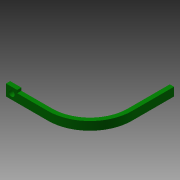
# Autodesk Inventor part: BackNetHookLeft
Saved by Autodesk Inventor 2014 SP1 (Build 180222100, 222)
## iProperties
Created: 2017-01-20
Part Number: BackNetHookLeft
Material: Generic
Document SubType Name: Modeling
Designer: danielsikar
Density: 1 g/cm^3
Appearance: Dark Green
Author: danielsikar
Autodesk Inventor part; units mm, degrees
ref_plane "YZ Plane" through (0, 0, 0) normal (1, 0, 0) x (0, 1, 0)
ref_plane "XZ Plane" through (0, 0, 0) normal (0, 1, 0) x (-1, 0, 0)
ref_plane "XY Plane" through (0, 0, 0) normal (0, 0, 1) x (1, 0, 0)
sketch "Sketch1" plane through (0, 0, 0) normal (0, 0, 1) x (1, 0, 0)
  line L0 (0, 0) -> (60, 0) construction
  line L1 (60, 0) -> (60, 60) construction
  line L2 (60, 60) -> (0, 60) construction
  line L3 (0, 3) -> (0, 0)
  line L4 (57, 60) -> (60, 60)
  line L5 (60, 60) -> (60, 30)
  line L6 (60, 0) -> (30, 0) construction
  line L7 (30, 0) -> (30, 30) construction
  line L8 (30, 30) -> (60, 30) construction
  line L9 (60, 30) -> (60, 0) construction
  arc A0 (30, 3) -> (57, 30) centre (30, 30) ccw
  line L10 (30, 3) -> (0, 3)
  line L11 (0, 0) -> (30, 0)
  line L12 (57, 30) -> (57, 60)
  line L13 (0, 60) -> (0, 30) construction
  line L14 (0, 3) -> (0, 0) construction
  arc A1 (30, 0) -> (60, 30) centre (30, 30) ccw
  arc A2 (30, 60) -> (0, 30) centre (30, 30) ccw
  dimension "d0" = 60
  dimension "d1" = 60
  dimension "d3" = 3
  dimension "d6" = 30
  constraints: 30 end point, 7 parallel, 6 point on circle, 3 centre point, 3 horizontal, 2 coincident, 2 perpendicular, 1 midpoint, 1 point on line
  measures "d0" distance of L2.end L1.end
  measures "d1" distance between parallel lines of L2 L0
  measures "d3" distance of L4.start L4.end
  measures "d6" distance of L5.end L7.end
extrude "Extrusion2" add sketch "Sketch1" along normal blind 6
sketch "Sketch2" plane through (0, 0, 6) normal (0, 0, 1) x (1, 0, 0)
  line L0 (30, 3) -> (0, 3) projected
  line L1 (0, 0) -> (8, 0)
  line L2 (8, 0) -> (8, 3)
  line L3 (8, 3) -> (0, 3)
  line L4 (0, 3) -> (0, 0)
  dimension "d10" = 8
  constraints: 8 end point, 2 parallel, 1 horizontal, 1 perpendicular, 1 point on line
  measures "d10" distance of L3.end L2.end
extrude "Extrusion3" add sketch "Sketch2" along normal blind 2
sketch "Sketch3" plane through (0, 3, 0) normal (0, 1, 0) x (1, 0, 0)
  circle A0 centre (4, -4) radius 2.15
  dimension "d13" = 4.3
  constraints: 1 centre point
  measures "d13" diameter of A0
extrude "Extrusion4" cut sketch "Sketch3" against normal through all
body "Solid2"
